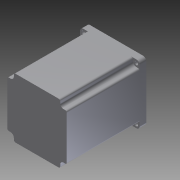
# Autodesk Inventor part: nema 23 frame size servo
Saved by Autodesk Inventor 2011 (Build 150239000, 239)
## iProperties
Created: 2013-11-18
Part Number: nema 23 frame size servo
Document SubType Name: Modeling
Designer: Devon
Density: 1 g/cm^3
Author: Devon
Autodesk Inventor part; units mm, degrees
ref_plane "YZ Plane" through (0, 0, 0) normal (1, 0, 0) x (0, 1, 0)
ref_plane "XZ Plane" through (0, 0, 0) normal (0, 1, 0) x (-1, 0, 0)
ref_plane "XY Plane" through (0, 0, 0) normal (0, 0, 1) x (1, 0, 0)
sketch "Sketch1" plane through (0, 0, 0) normal (0, 0, 1) x (1, 0, 0)
  line L0 (3.175, 0) -> (53.975, 0)
  line L1 (57.15, 3.175) -> (57.15, 53.975)
  line L2 (53.975, 57.15) -> (3.175, 57.15)
  line L3 (0, 53.975) -> (0, 3.175)
  arc A0 (3.175, 57.15) -> (0, 53.975) centre (3.175, 53.975) ccw
  arc A1 (57.15, 53.975) -> (53.975, 57.15) centre (53.975, 53.975) ccw
  arc A2 (53.975, 0) -> (57.15, 3.175) centre (53.975, 3.175) ccw
  arc A3 (0, 3.175) -> (3.175, 0) centre (3.175, 3.175) ccw
  point P0 (0, 0)
  point P1 (57.15, 57.15)
  point P2 (57.15, 0)
  point P3 (0, 57.15)
  dimension "d0" = 57.15
  dimension "d1" = 57.15
  dimension "d2" = 3.175
  constraints: 8 end point, 8 point on circle, 8 point on line, 8 tangent, 4 centre point, 3 equal radius, 2 parallel, 1 horizontal, 1 perpendicular
  measures "d0" distance of point (0, 57.15) point (57.15, 57.15)
  measures "d1" distance of point (57.15, 57.15) point (57.15, 0)
  measures "d2" radius of A0
extrude "Extrusion1" add sketch "Sketch1" along normal blind 6.35
sketch "Sketch2" plane through (0, 0, 6.35) normal (0, 0, 1) x (1, 0, 0)
  arc A0 (57.15, 53.975) -> (53.975, 57.15) centre (53.975, 53.975) ccw projected
  line L0 (3.175, 57.15) -> (53.975, 57.15) projected
  arc A1 (3.175, 57.15) -> (0, 53.975) centre (3.175, 53.975) ccw projected
  line L1 (0, 3.175) -> (0, 53.975) projected
  arc A2 (0, 3.175) -> (3.175, 0) centre (3.175, 3.175) ccw projected
  line L2 (53.975, 0) -> (3.175, 0) projected
  arc A3 (53.975, 0) -> (57.15, 3.175) centre (53.975, 3.175) ccw projected
  line L3 (57.15, 53.975) -> (57.15, 3.175) projected
  circle A4 centre (3.175, 53.975) radius 3.175
  circle A5 centre (53.975, 53.975) radius 3.175
  circle A6 centre (53.975, 3.175) radius 3.175
  circle A7 centre (3.175, 3.175) radius 3.175
  line L4 (6.35, 53.975) -> (6.35, 55.5498)
  line L5 (3.175, 50.8) -> (1.6002, 50.8)
  line L6 (50.8, 53.975) -> (50.8, 55.5498)
  line L7 (53.975, 50.8) -> (55.5498, 50.8)
  line L8 (53.975, 6.35) -> (55.5498, 6.35)
  line L9 (50.8, 3.175) -> (50.8, 1.6002)
  line L10 (6.35, 3.175) -> (6.35, 1.6002)
  line L11 (3.175, 6.35) -> (1.6002, 6.35)
  line L12 (7.9502, 57.15) -> (49.1998, 57.15)
  line L13 (57.15, 49.1998) -> (57.15, 7.9502)
  line L14 (49.1998, 0) -> (7.9502, 0)
  line L15 (0, 7.9502) -> (0, 49.1998)
  arc A8 (1.6002, 50.8) -> (0, 49.1998) centre (1.6002, 49.1998) ccw
  arc A9 (7.9502, 57.15) -> (6.35, 55.5498) centre (7.9502, 55.5498) ccw
  arc A10 (50.8, 55.5498) -> (49.1998, 57.15) centre (49.1998, 55.5498) ccw
  arc A11 (57.15, 49.1998) -> (55.5498, 50.8) centre (55.5498, 49.1998) ccw
  arc A12 (55.5498, 6.35) -> (57.15, 7.9502) centre (55.5498, 7.9502) ccw
  arc A13 (49.1998, 0) -> (50.8, 1.6002) centre (49.1998, 1.6002) ccw
  arc A14 (6.35, 1.6002) -> (7.9502, 0) centre (7.9502, 1.6002) ccw
  arc A15 (0, 7.9502) -> (1.6002, 6.35) centre (1.6002, 7.9502) ccw
  point P0 (0, 0)
  point P1 (6.35, 57.15)
  point P2 (0, 50.8)
  point P3 (50.8, 57.15)
  point P4 (57.15, 50.8)
  point P5 (57.15, 6.35)
  point P6 (50.8, 0)
  point P7 (6.35, 0)
  point P8 (0, 6.35)
  dimension "d5" = 1.6002
  constraints: 28 point on circle, 24 end point, 24 point on line, 24 tangent, 12 centre point, 7 equal radius, 7 perpendicular, 4 coincident, 3 parallel, 2 collinear
  measures "d5" radius of A8
extrude "Extrusion2" add sketch "Sketch2" along normal blind 69.85 contours L3 A12 L8 A6 L9 A13 L2 A14 L10 A7 L11 A15 L1 A8 L5 A4 L4 A9 L0 A10 L6 A5 L7 A11
sketch "Sketch3" plane through (0, 0, 0) normal (0, 0, -1) x (-1, 0, 0)
  arc A0 (-53.975, 57.15) -> (-57.15, 53.975) centre (-53.975, 53.975) ccw projected
  arc A1 (-57.15, 3.175) -> (-53.975, 0) centre (-53.975, 3.175) ccw projected
  arc A2 (-3.175, 0) -> (0, 3.175) centre (-3.175, 3.175) ccw projected
  arc A3 (0, 53.975) -> (-3.175, 57.15) centre (-3.175, 53.975) ccw projected
  circle A4 centre (-53.975, 53.975) radius 1.5875
  circle A5 centre (-3.175, 3.175) radius 1.5875
  circle A6 centre (-53.975, 3.175) radius 1.5875
  point P0 (0, 0)
  dimension "d8" = 3.175
  dimension "d10" = 3.175
  dimension "d11" = 3.175
  constraints: 3 centre point, 3 coincident
  measures "d8" diameter of A4
  measures "d10" diameter of A5
  measures "d11" diameter of A6
hole "Hole1" at (53.975, 53.975, 0) at (3.175, 53.975, 0) at (3.175, 3.175, 0) at (53.975, 3.175, 0) direction (0, 0, 1) diameter 3.175 depth 25.4 tip angle 118
sketch "Sketch4" plane through (0, 0, 0) normal (0, 0, -1) x (-1, 0, 0)
  circle A0 centre (-28.575, 28.575) radius 3.175
  point P0 (0, 0)
  dimension "d19" = 6.35
  constraints: 1 centre point
  measures "d19" diameter of A0
extrude "Extrusion3" add sketch "Sketch4" along normal blind 25.4
body "Solid1"
